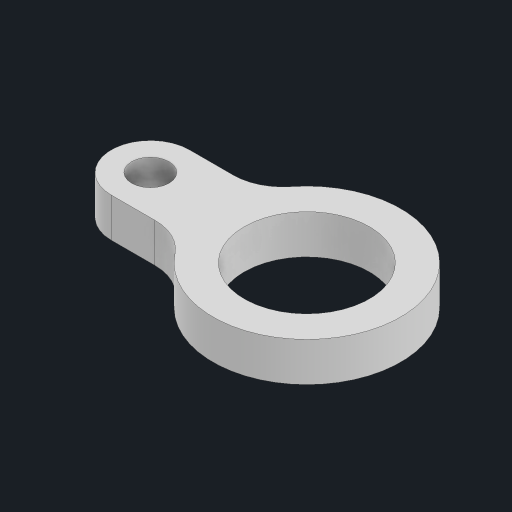
# Autodesk Inventor part: Capper Gate Linkage
Saved by Autodesk Inventor 2023.1 (Build 271208000, 208)
## iProperties
Created: 2023-05-23
Part Number: Capper Gate Linkage
Material: Generic
Document SubType Name: Modeling
Designer: Jarrett
Density: 1 g/cm^3
Appearance: Default
Author: Jarrett
Autodesk Inventor part; units mm, degrees
ref_plane "YZ Plane" through (0, 0, 0) normal (1, 0, 0) x (0, 1, 0)
ref_plane "XZ Plane" through (0, 0, 0) normal (0, 1, 0) x (-1, 0, 0)
ref_plane "XY Plane" through (0, 0, 0) normal (0, 0, 1) x (1, 0, 0)
sketch "Sketch1" plane through (0, 0, 0) normal (0, 1, 0) x (-1, 0, 0)
  circle A0 centre (0, 0) radius 8
  line L0 (0, 0) -> (20, 0) construction
  arc A1 (20, -5) -> (20, 5) centre (20, 0) ccw
  line L1 (20, -5) -> (10.9087, -5)
  arc A2 (10.9087, 5) -> (10.9087, -5) centre (0, 0) ccw
  line L2 (20, 5) -> (10.9087, 5)
  circle A3 centre (20, 0) radius 2.3916
  circle A4 centre (0, -2.25) radius 3.175
  point P0 (10.9087, -5)
  point P1 (10.9087, 5)
  dimension "d0" = 16
  dimension "d1" = 20
  dimension "d2" = 24
  dimension "d4" = 10
  dimension "d5" = 6.35
  dimension "d6" = 2.25
  constraints: 6 end point, 6 point on circle, 5 centre point, 4 coincident, 3 horizontal, 2 point on line, 2 tangent
  measures "d0" diameter of A0
  measures "d1" distance of L0.start L0.end
  measures "d2" diameter of A2
  measures "d4" diameter of A1
  measures "d5" diameter of A4
  measures "d6" distance of point (0, 0) A4.centre
extrude "Extrusion1" add sketch "Sketch1" along normal blind 5 contours L1 A2 L2 A1
fillet "Fillet1" radius 6.35 2 edges at (-10.9087, 2.5, -5) (-10.9087, 2.5, 5)
body "Solid1"
